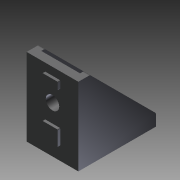
# Autodesk Inventor part: HBLFSNK5hblfsn5
Saved by Autodesk Inventor 2016 (Build 200138000, 138)
## iProperties
Category: PARTsolutions
Company: MISUMI
Created: 2016-06-25
Part Number: HBLFSNK5hblfsn5
Catalog Web Link: www.cadenas.de
Description: HBLFSN5, HBLFSNB5, HBLFSNM5, HBLFSNK5, HBLFSSW5, HBLFSSWB5, HBLFSDW5-Thin Reversal Brackets for Slot Width 6 Frames - For 20, 40mm Sections
Vendor: MISUMI
Document SubType Name: Modeling
Designer: psAdmin
Manufacturer: MISUMI
Mass: 16.727 g
Surface Area: 42.9533 cm^2
Volume: 6.19519 cm^3
Density: 2.7 g/cm^3
Material: アルミニウム 6061
Appearance: アルミニウム - フラット
PSOL_IDENT_0: {$CADENAS_DATA\23d-libs\misumi\metric\38_al_extrusions_blackets\5\hblfsn5.prj},243 {VTYP=3D},{NB=HBL
PSOL_IDENT_1: FSNK5hblfsn5},{LINA=HBLFSNK5hblfsn5},{NN=HBLFSN5, HBLFSNB5, HBLFSNM5, HBLFSNK5, HBLFSSW5, HBLFSSWB5,
PSOL_IDENT_2: HBLFSDW5},{DATE=17.07.2015 10:47:04},{GEOMDATE=28.01.2010 06:29:00},{VERSION=},{LINEID=40},{LINESUB
PSOL_IDENT_3: ID=-1},{WBVAR=ALT1,ALT2}  {NB=HBLFSNK5hblfsn5},{LINA=HBLFSNK5hblfsn5},{KT=1},{PN=HBLFSNK5},{TP=HBLFS
PSOL_IDENT_4: NK5},{NOH=1},{NOHV=2},{MAT=JIS-ADC12},{ST=-},{TYPE=HBLFSNK5},{FEAT=One Sided Slot Bracket},{ALT1=},{
PSOL_IDENT_5: ALT2=},{MASS=15},{AB=CBM5-10},{NOB=2},{AN=HNTT5-5},{NON=2},{AL=1176},{W=20},{H=30},{DP=30},{T=4.5},{
PSOL_IDENT_6: HDIS=8},{DPOS=12},{HH1=18},{BOLTX=0.0},{HV1=10},{BOLTY=0.0},{DIA=5.2},{ALT1OPT='','w/o C (Mounting H
PSOL_IDENT_7: oles for Cover)','-C','with C (Mounting Holes for Cover)'},{ALT2OPT= '' , 'w/o Set Applicable Bolt &
PSOL_IDENT_8: Nut' , '-SET' , 'with SET (Set Applicable Bolt & Nut)' , '-SST' , 'with SST (Stainless Steel Set Ap
PSOL_IDENT_9: plicable Bolt & Nut)' , '-SEP' , 'with SEP (Post Assembly Spring Nuts Set Applicable Bolt & Nut)' , '
PSOL_IDENT_10: -SSP' , 'with SSP (Post Assembly Spring Nuts, Stainless Steel Set Applicable Bolt & Nut)' },{R=1},{R
PSOL_IDENT_11: 1=0.3},{APOSV=0},{VER=1},{PR=1},{TT=1.0},{T1=2}
NN: HBLFSN5, HBLFSNB5, HBLFSNM5, HBLFSNK5, HBLFSSW5, HBLFSSWB5, HBLFSDW5
NT: Thin Reversal Brackets for Slot Width 6 Frames - For 20, 40mm Sections
NB: HBLFSNK5hblfsn5
NBSYN: $PN.hblfsn5
LINA: HBLFSNK5hblfsn5
PN: HBLFSNK5
TP: HBLFSNK5
MAT: JIS-ADC12
ST: -
FEAT: One Sided Slot Bracket
ALT1: w/o C (Mounting Holes for Cover)
ALT2: w/o Set Applicable Bolt & Nut
MASS: 15
AB: CBM5-10
NOB: 2
AN: HNTT5-5
NON: 2
AL: 1176
BOLTX: 0.0
BOLTY: 0.0
SUPPLIER: MISUMI
ARTICLENO: HBLFSNK5hblfsn5
BOMINFO: HBLFSNK5hblfsn5
CREATOR: CADENAS GmbH
Title: HBLFSNK5hblfsn5
Author: Cadenas PARTsolutions
Comments: Thin Reversal Brackets for Slot Width 6 Frames - For 20, 40mm Sections
Autodesk Inventor part; units mm, degrees
sketch "Sketch_15" plane through (0, 0, 0) normal (1, 0, 0) x (0, 1, 0)
  line L0 (0, 30) -> (0, 0)
  line L1 (0, 0) -> (30, 0)
  line L2 (30, 0) -> (30, 4.0858)
  arc A0 (30, 4.0858) -> (29.7071, 4.7929) centre (29, 4.0858) ccw
  line L3 (29.7071, 4.7929) -> (4.7929, 29.7071)
  arc A1 (4.7929, 29.7071) -> (4.0858, 30) centre (4.0858, 29) ccw
  line L4 (4.0858, 30) -> (0, 30)
  constraints: 10 end point, 4 point on circle, 2 centre point
extrude "Extrusion1" add sketch "Sketch_15" along normal mid plane 20
sketch "Sketch_16" plane through (0, 0, 0) normal (1, 0, 0) x (0, 1, 0)
  line L0 (2.9278, 34.5) -> (4.5, 4.5)
  line L1 (4.5, 4.5) -> (34.5, 4.5)
  line L2 (34.5, 4.5) -> (34.5, 34.5)
  line L3 (34.5, 34.5) -> (2.9278, 34.5)
  constraints: 8 end point
extrude "Extrusion2" cut sketch "Sketch_16" along normal mid plane 15
sketch "Sketch_17" plane through (0, 4.5, 0) normal (0, 1, 0) x (1, 0, 0)
  line L0 (-5.4209, -10.5) -> (-4.4687, -18.5299)
  arc A0 (-4.4687, -18.5299) -> (4.4687, -18.5299) centre (0, -18) ccw
  line L1 (4.4687, -18.5299) -> (5.4209, -10.5)
  line L2 (5.4209, -10.5) -> (-5.4209, -10.5)
  constraints: 6 end point, 2 point on circle, 1 centre point
extrude "Extrusion3" add sketch "Sketch_17" against normal blind 2.25
sketch "Sketch4" plane through (10, 0, 0) normal (0, 0, -1) x (-1, 0, 0)
  point P0 (10, 18)
hole "Hole1" at (0, 18, 0) direction (0, 0, 1) diameter 5.2 depth 4.5
sketch "Sketch5" plane through (10, 0, 0) normal (0, 0, -1) x (-1, 0, 0)
  point P0 (10, 10)
hole "Hole2" at (0, 10, 0) direction (0, 0, 1) diameter 5.2 depth 4.5
sketch "Sketch6" plane through (-10, 0, 30) normal (0, -1, 0) x (1, 0, 0)
  point P0 (10, -12)
hole "Hole3" at (0, 0, 18) direction (0, 1, 0) diameter 5.2 depth 4.5
sketch "Sketch_1" plane through (0, 0, 0) normal (0, 1, 0) x (-1, 0, 0)
  line L0 (10, 0) -> (10, 30)
  line L1 (10, 30) -> (-10, 30)
  line L2 (-10, 30) -> (-10, 0)
  line L3 (-10, 0) -> (10, 0)
  constraints: 8 end point
extrude "Extrusion4" add sketch "Sketch_1" against normal blind 1
sketch "Sketch_4" plane through (0, 0, 0) normal (0, 1, 0) x (-1, 0, 0)
  line L0 (10, 0) -> (10, 30)
  line L1 (10, 30) -> (-10, 30)
  line L2 (-10, 30) -> (-10, 0)
  line L3 (-10, 0) -> (10, 0)
  arc A0 (3, 10.7) -> (2.7, 11) centre (2.7, 10.7) ccw
  line L4 (2.7, 11) -> (-2.7, 11)
  arc A1 (-2.7, 11) -> (-3, 10.7) centre (-2.7, 10.7) ccw
  line L5 (-3, 10.7) -> (-3, 5.3)
  arc A2 (-3, 5.3) -> (-2.7, 5) centre (-2.7, 5.3) ccw
  line L6 (-2.7, 5) -> (2.7, 5)
  arc A3 (2.7, 5) -> (3, 5.3) centre (2.7, 5.3) ccw
  line L7 (3, 5.3) -> (3, 10.7)
  arc A4 (3, 26.7) -> (2.7, 27) centre (2.7, 26.7) ccw
  line L8 (2.7, 27) -> (-2.7, 27)
  arc A5 (-2.7, 27) -> (-3, 26.7) centre (-2.7, 26.7) ccw
  line L9 (-3, 26.7) -> (-3, 24.3)
  arc A6 (-3, 24.3) -> (-2.7, 24) centre (-2.7, 24.3) ccw
  line L10 (-2.7, 24) -> (2.7, 24)
  arc A7 (2.7, 24) -> (3, 24.3) centre (2.7, 24.3) ccw
  line L11 (3, 24.3) -> (3, 26.7)
  constraints: 24 end point, 16 point on circle, 8 centre point
extrude "Extrusion5" cut sketch "Sketch_4" against normal blind 1
ref_plane "bracket_to_bolt_XY" through (1, 10, 0) normal (0, 0, 1) x (1, 0, 0)
ref_plane "bracket_to_bolt_YZ" through (1, 10, 0) normal (1, 0, 0) x (0, 1, 0)
ref_plane "bracket_to_bolt_ZX" through (1, 10, 0) normal (0, 1, 0) x (0, 0, 1)
ref_plane "bracket_to_dummy_XY" through (0, 0, 0) normal (0, 1, 0) x (1, 0, 0)
ref_plane "bracket_to_dummy_YZ" through (0, 0, 0) normal (1, 0, 0) x (0, 0, -1)
ref_plane "bracket_to_dummy_ZX" through (0, 0, 0) normal (0, 0, -1) x (0, 1, 0)
ref_plane "to_bolt_4_7_base_XY" through (0, 4.5, 18) normal (0, 1, 0) x (1, 0, 0)
ref_plane "to_bolt_4_7_base_YZ" through (0, 4.5, 18) normal (1, 0, 0) x (0, 0, -1)
ref_plane "to_bolt_4_7_base_ZX" through (0, 4.5, 18) normal (0, 0, -1) x (0, 1, 0)
ref_plane "to_bolt_row_4_to_7_XY" through (0, 18, 4.5) normal (0, 0, 1) x (1, 0, 0)
ref_plane "to_bolt_row_4_to_7_YZ" through (0, 18, 4.5) normal (1, 0, 0) x (0, 1, 0)
ref_plane "to_bolt_row_4_to_7_ZX" through (0, 18, 4.5) normal (0, 1, 0) x (0, 0, 1)
ref_plane "to_nut_base_4_7_XY" through (0, -2, 18) normal (0, 1, 0) x (1, 0, 0)
ref_plane "to_nut_base_4_7_YZ" through (0, -2, 18) normal (1, 0, 0) x (0, 0, -1)
ref_plane "to_nut_base_4_7_ZX" through (0, -2, 18) normal (0, 0, -1) x (0, 1, 0)
ref_plane "to_nut_row_4_to_7_XY" through (0, 18, -2) normal (0, 0, 1) x (1, 0, 0)
ref_plane "to_nut_row_4_to_7_YZ" through (0, 18, -2) normal (1, 0, 0) x (0, 1, 0)
ref_plane "to_nut_row_4_to_7_ZX" through (0, 18, -2) normal (0, 1, 0) x (0, 0, 1)
body "Solid1"
